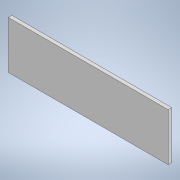
# Autodesk Inventor part: cab_L_B
Saved by Autodesk Inventor 2022 (Build 260153000, 153)
## iProperties
Created: 2023-03-05
Part Number: cab_L_B
Material: Generic
Document SubType Name: Modeling
Designer: Bunny
Density: 1 g/cm^3
Appearance: Default
Author: Bunny
Autodesk Inventor part; units mm, degrees
ref_plane "YZ Plane" through (0, 0, 0) normal (1, 0, 0) x (0, 1, 0)
ref_plane "XZ Plane" through (0, 0, 0) normal (0, 1, 0) x (-1, 0, 0)
ref_plane "XY Plane" through (0, 0, 0) normal (0, 0, 1) x (1, 0, 0)
sketch "Sketch1" plane through (0, 0, 0) normal (0, 0, 1) x (1, 0, 0)
  line L0 (-123.1394, 40.2933) -> (144.8606, 40.2933)
  line L1 (144.8606, 40.2933) -> (144.8606, -39.7067)
  line L2 (144.8606, -39.7067) -> (-123.1394, -39.7067)
  line L3 (-123.1394, -39.7067) -> (-123.1394, 40.2933)
  point P0 (0, 0)
  dimension "d0" = 268
  dimension "d1" = 80
  constraints: 8 end point, 2 parallel, 1 horizontal, 1 perpendicular
  measures "d0" distance of L0.start L0.end
  measures "d1" distance of L0.end L1.end
extrude "Extrusion1" add sketch "Sketch1" along normal blind 6
equation "\"d0\" = -2 * CornerOffset + BoxLength - 2 * SheetThickness"
equation "\"d1\" = BoxHeight"
equation "\"d2\" = SheetThickness"
equation "\"BoxHeight\" = 80"
equation "\"SheetThickness\" = 6"
equation "\"CornerOffset\" = 5"
equation "\"BoxLength\" = 290"
body "Solid1"
